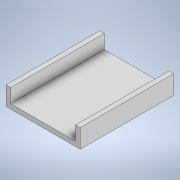
# Autodesk Inventor part: Blocker
Saved by Autodesk Inventor 2021 (Build 250183000, 183)
## iProperties
Created: 2021-01-09
Part Number: Blocker
Material: Generic
Document SubType Name: Modeling
Designer: User
Density: 1 g/cm^3
Appearance: Default
Author: User
Autodesk Inventor part; units mm, degrees
ref_plane "YZ Plane" through (0, 0, 0) normal (1, 0, 0) x (0, 1, 0)
ref_plane "XZ Plane" through (0, 0, 0) normal (0, 1, 0) x (-1, 0, 0)
ref_plane "XY Plane" through (0, 0, 0) normal (0, 0, 1) x (1, 0, 0)
sketch "Sketch1" plane through (0, 0, 0) normal (0, 0, 1) x (1, 0, 0)
  line L0 (0, 12.7) -> (0, 0)
  line L1 (0, 0) -> (50.292, 0)
  line L2 (50.292, 0) -> (50.292, 12.7)
  line L3 (3.175, 12.7) -> (3.175, 3.175)
  line L4 (3.175, 3.175) -> (47.117, 3.175)
  line L5 (47.117, 3.175) -> (47.117, 12.7)
  line L6 (3.175, 12.7) -> (0, 12.7)
  line L7 (47.117, 12.7) -> (50.292, 12.7)
  dimension "d2" = 50.292
  dimension "d3" = 12.7
  dimension "d4" = 12.7
  dimension "d5" = 3.175
  constraints: 16 end point, 2 perpendicular, 2 vertical, 1 collinear, 1 horizontal, 2 other
  measures "d2" distance between parallel lines of L2 L0
  measures "d3" distance of L1.end L2.end
  measures "d4" distance of L0.start L0.end
  measures "d5" distance between parallel lines of L0 L3
extrude "Extrusion1" add sketch "Sketch1" along normal blind 63.5
equation "\"d4\" = d3"
body "Solid1"
